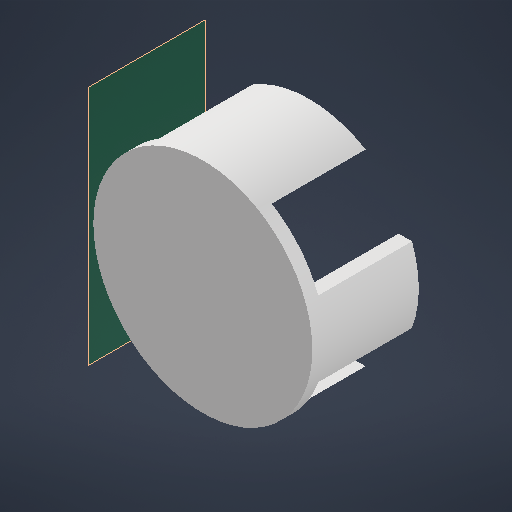
# Autodesk Inventor part: SistemLiberacion2
Saved by Autodesk Inventor 2026.1 (Build 301233000, 233)
## iProperties
Created: 2025-11-12
Part Number: SistemLiberacion2
Material: Genérico
Document SubType Name: Modeling
Designer: usuario
Density: 1 g/cm^3
Appearance: Valor por defecto
Author: usuario
Autodesk Inventor part; units mm, degrees
ref_plane "YZ Plane" through (0, 0, 0) normal (1, 0, 0) x (0, 1, 0)
ref_plane "XZ Plane" through (0, 0, 0) normal (0, 1, 0) x (-1, 0, 0)
ref_plane "XY Plane" through (0, 0, 0) normal (0, 0, 1) x (1, 0, 0)
sketch "Boceto1" plane through (0, 0, 0) normal (0, 0, 1) x (1, 0, 0)
  circle A0 centre (0, 0) radius 35
  dimension "d0" = 70
  constraints: 1 centre point, 1 coincident
  measures "d0" diameter of A0
extrude "Extrusión1" add sketch "Boceto1" along normal blind 34
shell "Vaciado1" thickness 4 removed faces 1 at (-1.9985, 11.019, 0)
ref_plane "Plano de trabajo2" through (-35, 0, 0) normal (-1, 0, 0) x (0, 0, -1)
ref_plane "Plano de trabajo1" through (-29.3614, 10, 16) normal (-1, 0, 0) x (0, 0, -1)
sketch "Boceto2" plane through (-35, 0, 0) normal (-1, 0, 0) x (0, 0, -1)
  line L0 (0, -31) -> (-30, -31) construction
  line L1 (0.1678, -31) -> (-30, -31) construction
  line L2 (-30, 31) -> (-30, -31) construction
  line L3 (0, 31) -> (-30, 31) construction
  line L4 (-30, -31) -> (0, -31) construction
  line L5 (0, -31) -> (0, 31) construction
  line L6 (0, 31) -> (-30, 31) construction
  line L7 (-30, 31) -> (-30, -31) construction
  line L8 (0, 35) -> (0, -35) construction
  line L9 (0, 31) -> (-30, -31) construction
  line L10 (-30, 31) -> (0, -31) construction
  line L11 (0, 30) -> (-30, 30)
  line L12 (-30, 30) -> (-30, 12)
  line L13 (-30, 12) -> (0, 12)
  line L14 (0, 12) -> (0, 30)
  line L15 (0, -12) -> (-30, -12)
  line L16 (-30, -12) -> (-30, -30)
  line L17 (-30, -30) -> (0, -30)
  line L18 (0, -30) -> (0, -12)
  point P0 (0, 0)
  point P1 (-15, 0)
  point P2 (-15, -30)
  point P3 (-15, 0)
  point P4 (-15, 30)
  dimension "d12" = 24
  dimension "d14" = 12
  dimension "d16" = 30
  dimension "d17" = 30
  constraints: 30 end point, 6 parallel, 6 point on line, 4 midpoint, 3 collinear, 3 horizontal, 3 perpendicular
  measures "d12" distance between parallel lines of L15 L13
  measures "d14" distance from line of point (-15, 0) L15
  measures "d16" distance of point (-15, 0) point (-15, 30)
  measures "d17" distance of point (-15, -30) point (-15, 0)
extrude "Extrusión2" cut sketch "Boceto2" against normal blind 86.75
equation "\"d14\" = 0.5 * d12"
equation "\"d17\" = d16"
